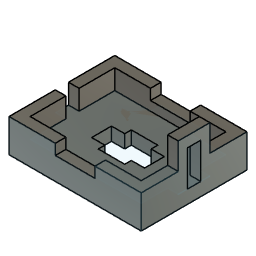
Sectional_Views_Model_Machine Block (Autodesk Fusion 360 design; units mm, degrees)
Autodesk Fusion 360 part; units mm, degrees
sketch "Sketch1" plane through (0, 0, 0) normal (0, 1, 0) x (1, 0, 0)
sketch "Sketch2" plane through (0, 0, 0) normal (0, 0, 1) x (1, 0, 0)
  line L0 (50, 0) -> (50, -40)
  line L1 (50, -40) -> (-50, -40)
  line L2 (-50, -40) -> (-50, 40)
  line L3 (-50, 40) -> (50, 40)
  line L4 (50, 40) -> (50, -40)
  constraint horizontal L1
  constraint vertical L2
  constraint horizontal L3
  constraint vertical L4
extrude "Extrude1" add sketch "Sketch2" along normal blind 10
sketch "Sketch3" plane through (0, 0, 10) normal (0, 0, 1) x (-1, 0, 0)
  line L0 (-50, -40) -> (50, -40)
  line L1 (50, -40) -> (50, 40)
  line L2 (50, 40) -> (-50, 40)
  line L3 (-50, 40) -> (-50, -40)
  line L4 (50, 40) -> (15, 40)
  line L5 (15, 40) -> (15, 32)
  line L6 (15, 32) -> (42, 32)
  line L7 (42, 32) -> (42, 5)
  line L8 (42, 5) -> (50, 5)
  line L9 (50, 5) -> (50, 40)
  dimension "d6" = 35
  dimension "d9" = 35
  constraint horizontal L4
  constraint vertical L5
  constraint horizontal L6
  constraint coincident L1.end L2.start
  constraint vertical L7
  constraint horizontal L8
  constraint vertical L9
  measures "d6" distance of L1.end L4.end
  measures "d9" distance of L1.end L8.end
extrude "Extrude2" add sketch "Sketch3" along normal blind 15 contours L1 L2 L4 L5 L6 L7 L8 L9
sketch "Sketch4" plane through (0, 0, 10) normal (0, 0, 1) x (-1, 0, 0)
  line L0 (15, 32) -> (15, 40)
  line L1 (15, 40) -> (-50, 40)
  line L2 (-50, 40) -> (-50, -40)
  line L3 (-50, -40) -> (50, -40)
  line L4 (50, -40) -> (50, 5)
  line L5 (50, 5) -> (42, 5)
  line L6 (42, 5) -> (42, 32)
  line L7 (42, 32) -> (15, 32)
  line L8 (15, 32) -> (-15, 32)
  line L9 (-15, 32) -> (-15, 40)
  line L10 (-15, 40) -> (15, 40)
  line L11 (15, 40) -> (15, 32)
  dimension "d12" = 30
  constraint horizontal L8
  constraint vertical L9
  constraint horizontal L10
  constraint vertical L11
  constraint coincident L0.start L7.end
  measures "d12" distance of L0.start L8.end
extrude "Extrude3" add sketch "Sketch4" along normal blind 7 contours L0 L1 L8 L9 L10 L11
sketch "Sketch5" plane through (0, 0, 10) normal (0, 0, 1) x (-1, 0, 0)
  line L0 (-15, 32) -> (-15, 40)
  line L1 (-15, 40) -> (-50, 40)
  line L2 (-50, 40) -> (-50, -40)
  line L3 (-50, -40) -> (50, -40)
  line L4 (50, -40) -> (50, 5)
  line L5 (50, 5) -> (42, 5)
  line L6 (42, 5) -> (42, 32)
  line L7 (42, 32) -> (-15, 32)
  line L8 (-15, 32) -> (-42, 32)
  line L9 (-50, 40) -> (-15, 40)
  line L10 (-15, 40) -> (-15, 32)
  line L11 (-42, 32) -> (-42, 12)
  line L12 (-42, 12) -> (-50, 12)
  line L13 (-50, 12) -> (-50, 40)
  dimension "d16" = 28
  constraint horizontal L8
  constraint horizontal L9
  constraint vertical L10
  constraint coincident L1.end L2.start
  constraint coincident L0.start L7.end
  constraint vertical L11
  constraint horizontal L12
  constraint vertical L13
  measures "d16" distance of L1.end L12.end
extrude "Extrude4" add sketch "Sketch5" along normal blind 15 contours L0 L1 L2 L8 L9 L10 L11 L12 L13
sketch "Sketch6" plane through (0, 0, 10) normal (0, 0, 1) x (-1, 0, 0)
  line L0 (-42, 12) -> (-50, 12)
  line L1 (-50, 12) -> (-50, -40)
  line L2 (-50, -40) -> (50, -40)
  line L3 (50, -40) -> (50, 5)
  line L4 (50, 5) -> (42, 5)
  line L5 (42, 5) -> (42, 32)
  line L6 (42, 32) -> (-42, 32)
  line L7 (-42, 32) -> (-42, 12)
  line L8 (42, -32) -> (42, -5)
  line L9 (42, -5) -> (50, -5)
  line L10 (50, -5) -> (50, -40)
  line L11 (50, -40) -> (15, -40)
  line L12 (15, -40) -> (15, -32)
  line L13 (15, -32) -> (42, -32)
  dimension "d19" = 35
  dimension "d20" = 35
  constraint vertical L8
  constraint horizontal L9
  constraint vertical L10
  constraint coincident L2.end L3.start
  constraint horizontal L11
  constraint vertical L12
  constraint horizontal L13
  measures "d19" distance of L2.end L9.end
  measures "d20" distance of L2.end L11.end
sketch "Sketch7" plane through (0, 0, 10) normal (0, 0, 1) x (-1, 0, 0)
  line L0 (-50, -40) -> (-42, -40)
  line L1 (-42, -32) -> (-42, -12)
  line L2 (-42, -12) -> (-50, -12)
  line L3 (-50, -12) -> (-50, -40)
  line L4 (-50, -40) -> (-15, -40)
  line L5 (-15, -40) -> (-15, -32)
  line L6 (-15, -32) -> (-42, -32)
  line L7 (-50, -32) -> (-50, -40)
  dimension "d22" = 8
  dimension "d23" = 28
  dimension "d24" = 35
  dimension "d25" = 8
  constraint horizontal L0
  constraint vertical L1
  constraint horizontal L2
  constraint vertical L3
  constraint horizontal L4
  constraint vertical L5
  constraint horizontal L6
  constraint vertical L7
  measures "d22" distance of L0.start L0.end
  measures "d23" distance of L0.start L2.end
  measures "d24" distance of L0.start L4.end
  measures "d25" distance of L0.start L7.start
extrude "Extrude5" add sketch "Sketch7" sketch "Sketch6" along normal blind 15 of sketch 2 contours L2 L3 L8 L9 L10 L11 L12 L13
sketch "Sketch8" plane through (0, 0, 10) normal (0, 0, 1) x (-1, 0, 0)
  line L0 (42, -5) -> (50, -5)
  line L1 (50, -5) -> (50, 5)
  line L2 (50, 5) -> (42, 5)
  line L3 (42, 5) -> (42, 32)
  line L4 (42, 32) -> (-42, 32)
  line L5 (-42, 32) -> (-42, 12)
  line L6 (-42, 12) -> (-50, 12)
  line L7 (-50, 12) -> (-50, -12)
  line L8 (-50, -12) -> (-42, -12)
  line L9 (-42, -12) -> (-42, -32)
  line L10 (-42, -32) -> (-15, -32)
  line L11 (-15, -32) -> (-15, -40)
  line L12 (-15, -40) -> (15, -40)
  line L13 (15, -40) -> (15, -32)
  line L14 (15, -32) -> (42, -32)
  line L15 (42, -32) -> (42, -5)
sketch "Sketch9" plane through (0, 0, 25) normal (0, 0, 1) x (-1, 0, 0)
  line L0 (-50, 12) -> (-42, 12)
  line L1 (-42, 12) -> (-42, 32)
  line L2 (-42, 32) -> (-15, 32)
  line L3 (-15, 32) -> (-15, 40)
  line L4 (-15, 40) -> (-50, 40)
  line L5 (-50, 40) -> (-50, 12)
sketch "Sketch10" plane through (0, 0, 10) normal (0, 0, 1) x (-1, 0, 0)
  line L0 (-50, 12) -> (-42, 12)
  line L1 (-42, 12) -> (-42, -12)
  line L2 (-42, -12) -> (-50, -12)
  line L3 (-50, -12) -> (-50, 12)
  constraint horizontal L0
  constraint vertical L1
  constraint horizontal L2
  constraint vertical L3
extrude "Extrude6" add sketch "Sketch10" along normal blind 35
sketch "Sketch11" plane through (0, 0, 10) normal (0, 0, 1) x (-1, 0, 0)
sketch "Sketch12" plane through (50, 0, 0) normal (1, 0, 0) x (0, 1, 0)
  line L0 (-40, 0) -> (40, 0)
  line L1 (40, 0) -> (40, 25)
  line L2 (40, 25) -> (12, 25)
  line L3 (12, 25) -> (12, 45)
  line L4 (12, 45) -> (-12, 45)
  line L5 (-12, 45) -> (-12, 25)
  line L6 (-12, 25) -> (-40, 25)
  line L7 (-40, 25) -> (-40, 0)
ref_plane "WorkPlane1" through (50, -12, 45) normal (1, 0, 0) x (0, 1, 0)
sketch "Sketch13" plane through (50, 0, 0) normal (1, 0, 0) x (0, 1, 0)
  line L0 (0, 37) -> (5, 37)
  line L1 (5, 37) -> (-5, 37)
  line L2 (-5, 37) -> (-5, 10)
  line L3 (-5, 10) -> (5, 10)
  line L4 (5, 10) -> (5, 37)
  dimension "d31" = 5
  dimension "d32" = 27
  constraint horizontal L1
  constraint vertical L2
  constraint horizontal L3
  constraint vertical L4
  measures "d31" distance of L0.start L0.end
  measures "d32" distance of L0.end L3.end
extrude "Extrude7" cut sketch "Sketch13" against normal blind 200
sketch "Sketch14" plane through (0, 0, 10) normal (0, 0, 1) x (-1, 0, 0)
  line L0 (-20, 0) -> (-20, 7.5)
  line L1 (20, 0) -> (20, -7.5)
  line L2 (-20, -7.5) -> (-20, 0)
  line L3 (10, -7.5) -> (10, -12.5)
  line L4 (10, -12.5) -> (-10, -12.5)
  line L5 (-10, -12.5) -> (-10, -7.5)
  line L6 (20, -7.5) -> (10, -7.5)
  line L7 (-10, -7.5) -> (-20, -7.5)
  line L8 (10, 12.5) -> (-10, 12.5)
  line L9 (10, 7.5) -> (10, 12.5)
  line L10 (20, 7.5) -> (10, 7.5)
  line L11 (20, 0) -> (20, 7.5)
  line L12 (-10, 12.5) -> (-10, 7.5)
  line L13 (-10, 7.5) -> (-20, 7.5)
  line L14 (-20, 7.5) -> (-20, 0)
  dimension "d35" = 20
  dimension "d36" = 7.5
  dimension "d37" = 15
  dimension "d40" = 20
  dimension "d41" = 5
  constraint vertical L1
  constraint horizontal L6
  constraint vertical L2
  constraint coincident L5.end L6
  constraint vertical L3
  constraint horizontal L4
  constraint vertical L5
  constraint collinear L6 L7
  measures "d35" distance of origin L0.start
  measures "d36" distance of L0.start L0.end
  measures "d37" distance of L0.end L2.start
  measures "d40" distance of L5.end L3.start
  measures "d41" distance of L5.end L4.end
extrude "Extrude8" cut sketch "Sketch14" against normal blind 100
sketch "Sketch15" plane through (0, -40, 0) normal (0, -1, 0) x (1, 0, 0)
  line L0 (-50, 0) -> (50, 0)
  line L1 (50, 0) -> (50, 25)
  line L2 (50, 25) -> (15, 25)
  line L3 (15, 25) -> (15, 17)
  line L4 (15, 17) -> (-15, 17)
  line L5 (-15, 17) -> (-15, 25)
  line L6 (-15, 25) -> (-50, 25)
  line L7 (-50, 25) -> (-50, 0)
sketch "Sketch16" plane through (0, 0, 10) normal (0, 0, 1) x (-1, 0, 0)
sketch "Sketch17" plane through (0, 0, 10) normal (0, 0, 1) x (-1, 0, 0)
  line L0 (-15, -32) -> (15, -32)
  line L1 (15, -32) -> (15, -40)
  line L2 (15, -40) -> (-15, -40)
  line L3 (-15, -40) -> (-15, -32)
  constraint horizontal L0
  constraint vertical L1
  constraint horizontal L2
  constraint vertical L3
extrude "Extrude9" add sketch "Sketch17" along normal blind 7
